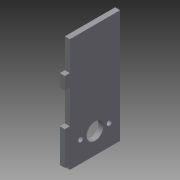
# Autodesk Inventor part: Motor support
Saved by Autodesk Inventor 2015 (Build 190159000, 159)
## iProperties
Created: 2014-08-11
Part Number: Motor support
Material: Generic
Document SubType Name: Modeling
Designer: karl
Density: 1 g/cm^3
Appearance: Default
Author: karl
Autodesk Inventor part; units mm, degrees
ref_plane "YZ Plane" through (0, 0, 0) normal (1, 0, 0) x (0, 1, 0)
ref_plane "XZ Plane" through (0, 0, 0) normal (0, 1, 0) x (-1, 0, 0)
ref_plane "XY Plane" through (0, 0, 0) normal (0, 0, 1) x (1, 0, 0)
sketch "Sketch1" plane through (0, 0, 0) normal (1, 0, 0) x (0, 1, 0)
  line L0 (15, 52) -> (-15, 52)
  line L1 (-15, 52) -> (-15, -12.5)
  line L2 (-15, -12.5) -> (15, -12.5)
  line L3 (15, -12.5) -> (15, 52)
  line L4 (-15, 10) -> (-18, 10)
  line L5 (-18, 10) -> (-18, -10)
  line L6 (-18, -10) -> (-15, -10)
  line L7 (-15, -10) -> (-15, 10)
  line L8 (-15, 42.5) -> (-18, 42.5)
  line L9 (-18, 42.5) -> (-18, 35)
  line L10 (-18, 35) -> (-15, 35)
  line L11 (-15, 35) -> (-15, 42.5)
  point P0 (0, 0)
  point P1 (0, -12.5)
  point P2 (-18, 0)
  dimension "d0" = 52
  dimension "d1" = 12.5
  dimension "d2" = 3
  dimension "d3" = 20
  dimension "d4" = 7.5
  dimension "d5" = 25
  dimension "d8" = 30
  constraints: 24 end point, 6 parallel, 3 horizontal, 3 perpendicular, 2 midpoint, 2 point on line, 1 collinear, 1 horizontal alignment, 1 vertical alignment
  measures "d0" distance from line of L0 point (0, 0)
  measures "d1" distance from line of L2 point (0, 0)
  measures "d2" distance of L6.end L5.end
  measures "d3" distance of L5.end L4.end
  measures "d4" distance of L9.end L8.end
  measures "d5" distance between parallel lines of L4 L10
  measures "d8" distance between parallel lines of L1 L3
extrude "Extrusion1" add sketch "Sketch1" along normal blind 3
sketch "Sketch2" plane through (3, 0, 0) normal (1, 0, 0) x (0, 0, -1)
  circle A0 centre (0, -2.5) radius 5
  circle A1 centre (0, 6) radius 1.5
  circle A2 centre (0, -11) radius 1.5
  line L0 (-10, -18) -> (10, -18) projected
  line L1 (-35, -15) -> (-10, -15) projected
  point P0 (0, -18)
  dimension "d9" = 10
  dimension "d10" = 3
  dimension "d11" = 3
  dimension "d12" = 17
  dimension "d13" = 8.5
  dimension "d20" = 12.5
  constraints: 3 centre point, 3 vertical alignment, 1 coincident, 1 midpoint
  measures "d9" diameter of A0
  measures "d10" diameter of A1
  measures "d11" diameter of A2
  measures "d12" distance of A1.centre A2.centre
  measures "d13" distance of point (0, -2.5) A2.centre
  measures "d20" distance from line of L1 point (0, -2.5)
extrude "Extrusion2" cut sketch "Sketch2" against normal blind 3
sketch "Sketch3" plane through (3, 0, 0) normal (1, 0, 0) x (0, 0, -1)
  line L0 (-52, 15) -> (-52, -15) projected
  line L1 (-52, 5) -> (-55, 5)
  line L2 (-55, 5) -> (-55, -5)
  line L3 (-55, -5) -> (-52, -5)
  line L4 (-52, -5) -> (-52, 5)
  point P0 (0, 0)
  point P1 (-55, 0)
  dimension "d16" = 3
  dimension "d17" = 10
  constraints: 8 end point, 2 parallel, 1 horizontal, 1 horizontal alignment, 1 midpoint, 1 perpendicular, 1 point on line
  measures "d16" distance of L3.end L2.end
  measures "d17" distance of L2.end L1.end
extrude "Extrusion3" add sketch "Sketch3" against normal blind 3
equation "\"d13\" = 0.5 * d12"
body "Solid1"
